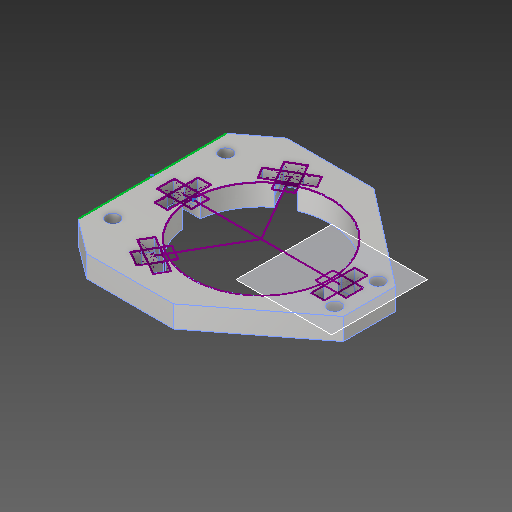
# Autodesk Inventor part: trackball-base
Saved by Autodesk Inventor 2018 (Build 220112000, 112)
## iProperties
Created: 2018-06-15
Part Number: trackball-base
Material: アルミニウム 6061
Document SubType Name: モデリング
Designer: NaMACHAN
Density: 2.7 g/cm^3
Appearance: アルミニウム - フラット
Mass: 12.2797 g
Surface Area: 37.8361 cm^2
Volume: 4.54805 cm^3
Sheet Metal Rule: Default
Author: NaMACHAN
Autodesk Inventor part; units mm, degrees
ref_plane "YZ Plane" through (0, 0, 0) normal (1, 0, 0) x (0, 1, 0)
ref_plane "XZ Plane" through (0, 0, 0) normal (0, 1, 0) x (-1, 0, 0)
ref_plane "XY Plane" through (0, 0, 0) normal (0, 0, 1) x (1, 0, 0)
sketch "スケッチ1" plane through (0, 0, 0) normal (0, 1, 0) x (-1, 0, 0)
  line L0 (33.3103, -23) -> (13.3103, -23)
  line L1 (13.3103, -23) -> (-8.6897, -6)
  line L2 (-8.6897, -6) -> (-8.6897, 6)
  line L3 (-8.6897, 6) -> (13.3103, 23)
  line L4 (13.3103, 23) -> (33.3103, 23)
  line L5 (-8.6897, -6) -> (33.3103, 23) construction
  line L6 (33.3103, -23) -> (-8.6897, 6) construction
  line L7 (33.3103, -23) -> (41.3103, -17)
  line L8 (41.3103, -17) -> (41.3103, 17)
  line L9 (41.3103, 17) -> (33.3103, 23)
  point P0 (0, 0)
  point P1 (0, 0)
  dimension "d1" = 46
  dimension "d50" = 20
  dimension "d51" = 20
  dimension "d52" = 17
  dimension "d53" = 17
  dimension "d72" = 8
  dimension "d73" = 6
  dimension "d74" = 6
  dimension "d75" = 50
  constraints: 20 end point, 2 point on line, 2 vertical alignment, 1 coincident, 1 horizontal, 1 parallel, 1 perpendicular, 1 vertical
  measures "d1" distance of L4.end L0.start
  measures "d50" distance of L3.end L4.end
  measures "d51" distance of L0.start L0.end
  measures "d52" vertical distance of L1.end L0.end
  measures "d53" vertical distance of L2.end L3.end
  measures "d72" distance from line of L8 L0.start
  measures "d73" vertical distance of L0.start L7.end
  measures "d74" vertical distance of L4.end L8.end
  measures "d75" distance between parallel lines of L2 L8
extrude "押し出し5" add sketch "スケッチ1" along normal blind 5
ref_plane "作業平面2" through (0, 5, 0) normal (0, 1, 0) x (1, 0, 0)
sketch "スケッチ4" plane through (0, 5, 0) normal (0, 1, 0) x (1, 0, 0)
  line L0 (-16.3103, 0) -> (-25.3103, -15.5885)
  line L1 (-25.3103, -15.5885) -> (-16.3103, 0)
  line L2 (-25.3103, 15.5885) -> (-16.3103, 0)
  line L3 (-16.3103, 0) -> (1.6897, 0)
  line L4 (-20.2302, -16.7894) -> (-28.8905, -11.7894)
  line L5 (-28.8905, -11.7894) -> (-30.3905, -14.3875)
  line L6 (-30.3905, -14.3875) -> (-21.7302, -19.3875)
  line L7 (-21.7302, -19.3875) -> (-20.2302, -16.7894)
  line L8 (-20.2302, -16.7894) -> (-30.3905, -14.3875) construction
  line L9 (-28.8905, -11.7894) -> (-21.7302, -19.3875) construction
  line L10 (-20.2302, 16.7894) -> (-28.8905, 11.7894)
  line L11 (-28.8905, 11.7894) -> (-30.3905, 14.3875)
  line L12 (-30.3905, 14.3875) -> (-21.7302, 19.3875)
  line L13 (-21.7302, 19.3875) -> (-20.2302, 16.7894)
  line L14 (-20.2302, 16.7894) -> (-30.3905, 14.3875) construction
  line L15 (-28.8905, 11.7894) -> (-21.7302, 19.3875) construction
  line L16 (-25.2924, -11.5574) -> (-28.7924, -17.6195)
  line L17 (-28.7924, -17.6195) -> (-25.3283, -19.6195)
  line L18 (-25.3283, -19.6195) -> (-21.8283, -13.5574)
  line L19 (-21.8283, -13.5574) -> (-25.2924, -11.5574)
  line L20 (-25.2924, -11.5574) -> (-25.3283, -19.6195) construction
  line L21 (-28.7924, -17.6195) -> (-21.8283, -13.5574) construction
  line L22 (-29.0424, 18.0526) -> (-25.0424, 11.1244)
  line L23 (-25.0424, 11.1244) -> (-21.5783, 13.1244)
  line L24 (-21.5783, 13.1244) -> (-25.5783, 20.0526)
  line L25 (-25.5783, 20.0526) -> (-29.0424, 18.0526)
  line L26 (-29.0424, 18.0526) -> (-21.5783, 13.1244) construction
  line L27 (-25.0424, 11.1244) -> (-25.5783, 20.0526) construction
  line L28 (3.1897, -5) -> (3.1897, 5)
  line L29 (3.1897, 5) -> (0.1897, 5)
  line L30 (0.1897, 5) -> (0.1897, -5)
  line L31 (0.1897, -5) -> (3.1897, -5)
  line L32 (3.1897, -5) -> (0.1897, 5) construction
  line L33 (3.1897, 5) -> (0.1897, -5) construction
  line L34 (5.1897, 2) -> (-1.8103, 2)
  line L35 (-1.8103, 2) -> (-1.8103, -2)
  line L36 (-1.8103, -2) -> (5.1897, -2)
  line L37 (5.1897, -2) -> (5.1897, 2)
  line L38 (5.1897, 2) -> (-1.8103, -2) construction
  line L39 (-1.8103, 2) -> (5.1897, -2) construction
  circle A0 centre (-16.3103, 0) radius 16
  line L40 (-41.3103, 17) -> (-41.3103, -17) projected
  line L41 (-16.3103, 0) -> (-34.3103, 0)
  line L42 (-32.8103, -5) -> (-35.8103, -5)
  line L43 (-35.8103, -5) -> (-35.8103, 5)
  line L44 (-35.8103, 5) -> (-32.8103, 5)
  line L45 (-32.8103, 5) -> (-32.8103, -5)
  line L46 (-32.8103, -5) -> (-35.8103, 5) construction
  line L47 (-35.8103, -5) -> (-32.8103, 5) construction
  line L48 (-38.3103, -2) -> (-30.3103, -2)
  line L49 (-30.3103, -2) -> (-30.3103, 2)
  line L50 (-30.3103, 2) -> (-38.3103, 2)
  line L51 (-38.3103, 2) -> (-38.3103, -2)
  line L52 (-38.3103, -2) -> (-30.3103, 2) construction
  line L53 (-30.3103, -2) -> (-38.3103, 2) construction
  point P0 (-31.7241, 0)
  point P1 (-41.3103, 0)
  point P2 (-41.3103, 0)
  dimension "d8" = 120
  dimension "d9" = 120
  dimension "d10" = 18
  dimension "d11" = 18
  dimension "d12" = 18
  dimension "d13" = 4
  dimension "d14" = 4
  dimension "d15" = 4
  dimension "d16" = 7
  dimension "d17" = 3
  dimension "d18" = 10
  dimension "d19" = 8
  dimension "d20" = 10
  dimension "d21" = 3
  dimension "d22" = 10
  dimension "d23" = 3
  dimension "d24" = 7
  dimension "d29" = 32
  dimension "d79" = 25
  dimension "d121" = 18
  dimension "d122" = 4
  dimension "d123" = 8
  dimension "d124" = 3
  dimension "d125" = 10
  constraints: 106 end point, 17 equal length, 17 midpoint, 14 perpendicular, 4 horizontal, 3 horizontal alignment, 1 centre point, 1 coincident
  measures "d8" angle of L2 L3
  measures "d9" angle of L0 L3
  measures "d10" distance of L0.start L0.end
  measures "d11" distance of L2.start L0.start
  measures "d12" distance of L0.start L3.end
  measures "d13" distance of L18.end L16.start
  measures "d14" distance of L22.end L23.end
  measures "d15" distance of L34.end L35.end
  measures "d16" distance of L17.end L18.end
  measures "d17" distance of L4.end L5.end
  measures "d18" distance of L5.end L6.end
  measures "d19" distance of L22.start L22.end
  measures "d20" distance of L11.end L12.end
  measures "d21" distance of L12.end L10.start
  measures "d22" distance of L28.start L28.end
  measures "d23" distance of L28.end L29.end
  measures "d24" distance between parallel lines of L35 L37
  measures "d29" diameter of A0
  measures "d79" distance from line of L40 L0.start
  measures "d121" distance of L41.start L41.end
  measures "d122" distance of L48.end L49.end
  measures "d123" distance of L49.end L50.end
  measures "d124" distance of L43.end L44.end
  measures "d125" distance of L42.end L43.end
extrude "押し出し2" cut sketch "スケッチ4" against normal blind 10 contours L19 L18 A0 L0 | L0 A0 L16 L19 | L23 L22 A0 L2 | L2 A0 L24 L23 | L35 L34 A0 L3 | L3 A0 L36 L35 | L49 L48 A0 L41 | L41 A0 L50 L49 | A0 L18 L4 L0 | L0 L4 L16 A0 | A0 L22 L10 L2 | L2 L10 L24 A0 | A0 L34 L30 L3 | L3 L30 L36 A0 | L41 L45 L50 A0 | A0 L48 L45 L41 | L4 L18 L6 L16 | L10 L22 L12 L24 | L30 L34 L28 L36 | L45 L48 L43 L50 | L18 L17 L16 L6 | L12 L22 L25 L24 | L34 L37 L36 L28 | L43 L48 L51 L50
extrude "押し出し3" cut sketch "スケッチ4" against normal blind 3 contours L4 L18 L6 L16 | L10 L22 L12 L24 | L30 L34 L28 L36 | L45 L48 L43 L50 | L4 L7 L6 L18 | L16 L6 L5 L4 | L24 L12 L13 L10 | L10 L11 L12 L22 | L30 L29 L28 L34 | L36 L28 L31 L30 | L50 L43 L44 L45 | L45 L42 L43 L48
extrude "押し出し4" cut sketch "スケッチ4" against normal blind 10 contours L3 L35 L36 A0 L18 L19 L0 | L41 L49 L50 A0 L22 L23 L2 | L2 L23 L24 A0 L34 L35 L3 | L0 L19 L16 A0 L48 L49 L41 | L19 L18 A0 L0 | L0 A0 L16 L19 | L23 L22 A0 L2 | L2 A0 L24 L23 | L35 L34 A0 L3 | L3 A0 L36 L35 | L49 L48 A0 L41 | L41 A0 L50 L49
ref_plane "作業平面1" through (0, 5, 0) normal (0, 1, 0) x (1, 0, 0)
sketch "スケッチ6" plane through (0, 5, 0) normal (0, 1, 0) x (1, 0, 0)
  line L0 (8.6897, -6) -> (8.6897, 6) projected
  line L1 (-33.3103, -23) -> (-13.3103, -23) projected
  line L2 (-13.3103, 23) -> (-33.3103, 23) projected
  point P0 (0, 0)
  point P1 (5.6897, 5)
  point P2 (5.6897, -5)
  point P3 (-37.3103, 13)
  point P4 (-37.3103, -13)
  dimension "d58" = 1
  dimension "d59" = 1
  dimension "d60" = 24
  dimension "d80" = 3
  dimension "d81" = 10
  dimension "d82" = 10
  constraints: 1 vertical alignment
  measures "d58" vertical distance of L0.end point (5.69, 5)
  measures "d59" vertical distance of L0.start point (5.69, -5)
  measures "d60" horizontal distance of L1.end point (-37.31, -13)
  measures "d80" distance from line of L0 point (5.69, 5)
  measures "d81" distance from line of point (-37.31, -13) L1
  measures "d82" distance from line of point (-37.31, 13) L2
hole "穴2" at (5.6897, 5, -5) at (5.6897, 5, 5) at (-37.3103, 5, -13) at (-37.3103, 5, 13) direction (0, -1, 0) diameter 3 end through all
equation "\"d11\" = d10"
equation "\"d12\" = d10"
equation "\"d14\" = d13"
equation "\"d15\" = d13"
equation "\"d20\" = d18"
equation "\"d21\" = d17"
equation "\"d22\" = d18"
equation "\"d23\" = d17"
equation "\"d24\" = d16"
equation "\"d121\" = d11"
equation "\"d122\" = d14"
equation "\"d123\" = d19"
equation "\"d124\" = d21"
equation "\"d125\" = d20"
equation "\"d66\" = Thickness"
equation "\"BendRadius\" = Thickness"
equation "\"BendReliefWidth\" = Thickness"
equation "\"BendReliefDepth\" = 0.5 * Thickness"
equation "\"TransitionRadius\" = BendRadius"
equation "\"JacobiRadiusSize\" = Thickness"
equation "\"GapSize\" = Thickness"
equation "\"d2\" = Thickness"
equation "\"Thickness\" = 5"
